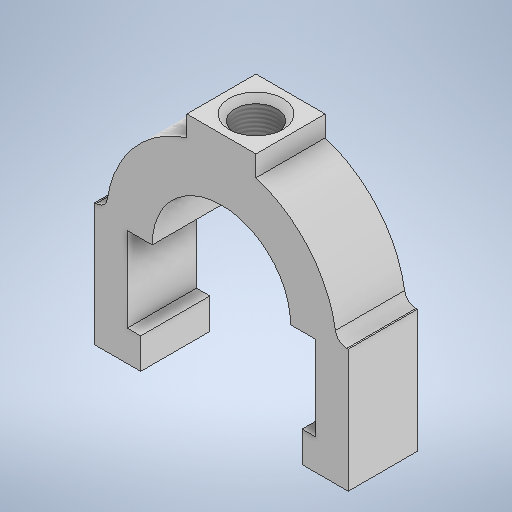
# Autodesk Inventor part: picovina
Saved by Autodesk Inventor 2025 (Build 290162000, 162)
## iProperties
Created: 2025-04-24
Part Number: picovina
Material: Všeobecné
Document SubType Name: Modeling
Designer: jakub
Density: 1 g/cm^3
Appearance: Výchozí
Author: jakub
Autodesk Inventor part; units mm, degrees
ref_plane "YZ Plane" through (0, 0, 0) normal (1, 0, 0) x (0, 1, 0)
ref_plane "XZ Plane" through (0, 0, 0) normal (0, 1, 0) x (-1, 0, 0)
ref_plane "XY Plane" through (0, 0, 0) normal (0, 0, 1) x (1, 0, 0)
sketch "Sketch1" plane through (0, 0, 0) normal (0, 0, 1) x (1, 0, 0)
  line L0 (0, 0) -> (-12, 0)
  line L1 (-12, 0) -> (-12, 32)
  line L2 (0, 0) -> (0, 8)
  line L3 (0, 8) -> (-3.5, 8)
  line L4 (-3.5, 8) -> (-3.5, 30)
  line L5 (-3.5, 30) -> (3, 30)
  line L6 (-12, 32) -> (-11.619, 32)
  arc A0 (-11.619, 32) -> (-8.6536, 34.5455) centre (-11.619, 35) ccw
  arc A1 (39, 30) -> (3, 30) centre (21, 30) ccw
  line L7 (3, 30) -> (-3.5, 30)
  line L8 (-3.5, 30) -> (3, 30)
  line L9 (12, 45.5885) -> (12, 64)
  line L10 (21, 64) -> (12, 64)
  line L11 (42, 0) -> (54, 0)
  line L12 (54, 0) -> (54, 32)
  line L13 (42, 0) -> (42, 8)
  line L14 (42, 8) -> (45.5, 8)
  line L15 (45.5, 8) -> (45.5, 30)
  line L16 (45.5, 30) -> (39, 30)
  line L17 (54, 32) -> (53.619, 32)
  arc A2 (50.6536, 34.5455) -> (53.619, 32) centre (53.619, 35) ccw
  arc A3 (39, 30) -> (3, 30) centre (21, 30) ccw
  line L18 (39, 30) -> (45.5, 30)
  line L19 (45.5, 30) -> (39, 30)
  line L20 (30, 45.5885) -> (30, 64)
  line L21 (21, 64) -> (30, 64)
  arc A4 (50.6536, 34.5455) -> (30, 58.6182) centre (21, 30) ccw
  arc A5 (12, 58.6182) -> (-8.6536, 34.5455) centre (21, 30) ccw
  arc A6 (50.6536, 34.5455) -> (30, 58.6182) centre (21, 30) ccw
  arc A7 (12, 58.6182) -> (-8.6536, 34.5455) centre (21, 30) ccw
  point P0 (51, 30)
  point P1 (12, 30)
  point P2 (-9, 30)
  point P3 (30, 30)
  point P4 (39, 30)
  constraints: 44 end point, 18 point on circle, 8 centre point, 5 perpendicular, 3 horizontal, 3 point on line, 2 coincident, 1 tangent, 1 vertical
extrude "Extrusion1" add sketch "Sketch1" along normal mid plane 18
sketch "Sketch2" plane through (12, 64, 9) normal (0, 1, 0) x (1, 0, 0)
  line L0 (0, 18) -> (0, 0)
  line L1 (0, 0) -> (9, 0)
  line L2 (27, 0) -> (-9, 0)
  line L3 (9, 0) -> (9, 9)
  point P0 (-12, 9)
  dimension "d17" = 9
  dimension "d18" = 9
  constraints: 8 end point, 1 midpoint
  measures "d17" distance of L0.end L1.end
  measures "d18" distance of L1.end L3.end
hole "Hole1" at (21, 64, 0) direction (0, -1, 0) diameter 10.917 depth 29.1 countersink diameter 14 countersink angle 90 thread size "M12x1" class "6H" standard "ISO Metric profile"
body "Solid1"
